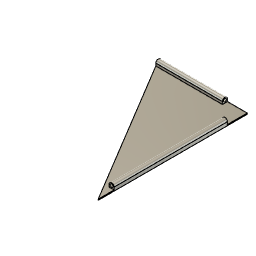
SE-RU v1 (Autodesk Fusion 360 design; units mm, degrees)
Autodesk Fusion 360 part; units mm, degrees
sketch "スケッチ1" plane through (0, 0, 0) normal (0, 1, 0) x (1, 0, 0)
  line L0 (0, 0) -> (0, -150)
  line L1 (0, 0) -> (-90, 0)
  line L2 (-90, 0) -> (0, -150)
  dimension "d1" = 150
  dimension "d2" = 90
  constraint coincident L0.start L1.start
  constraint vertical L0
  constraint perpendicular L0 L1
  measures "d1" distance of L0.start L0.end
  measures "d2" distance of L0.start L1.end
extrude "押し出し1" add sketch "スケッチ1" along normal blind 1
ref_plane "作業平面1" through (-45, 0.5, 20) normal (0, 0, -1) x (-1, 0, 0)
sketch "スケッチ2" plane through (0, 0, 20) normal (0, 0, -1) x (-1, 0, 0)
  circle A0 centre (2.5, 3.5) radius 1.5
  line L0 (0, 1) -> (90, 1)
  line L1 (0, 1.75) -> (0, 22.5)
  circle A1 centre (2.5, 3.5) radius 2.5
  line L2 (5, 3.5) -> (5, 1)
  line L3 (0, 3.5) -> (0, 1)
  dimension "d6" = 3
  dimension "d7" = 1
  constraint tangent L0 A1
  constraint tangent L1 A1
  constraint coincident A1 L2.start
  constraint coincident L0 L2.end
  constraint tangent A1 L2
  constraint perpendicular L0 L2
  constraint coincident A1 L3.start
  constraint coincident L1 L3.start
  constraint coincident L0.start L3.end
  measures "d6" diameter of A0
extrude "押し出し2" add sketch "スケッチ2" against normal blind 114
ref_plane "作業平面2" through (-20, 1.75, 75) normal (1, 0, 0) x (0, 0, -1)
sketch "スケッチ3" plane through (-20, 0, 0) normal (1, 0, 0) x (0, 0, -1)
  circle A0 centre (-2.5, 3.5) radius 1.5
  circle A1 centre (-2.5, 3.5) radius 2.5
  line L0 (-20, 1) -> (0, 1)
  line L1 (0, 1.75) -> (0, 22.5)
  line L2 (0, 3.5) -> (0, 1)
  line L3 (-5, 3.5) -> (-5, 1)
  dimension "d11" = 3
  dimension "d12" = 1
  constraint tangent A1 L0
  constraint tangent A1 L1
  constraint coincident A1 L2.start
  constraint coincident L0.end L2.end
  constraint perpendicular L0 L2
  constraint coincident A1 L3.start
  constraint coincident L0 L3.end
  constraint perpendicular L0 L3
  measures "d11" diameter of A0
extrude "押し出し3" add sketch "スケッチ3" against normal blind 67
